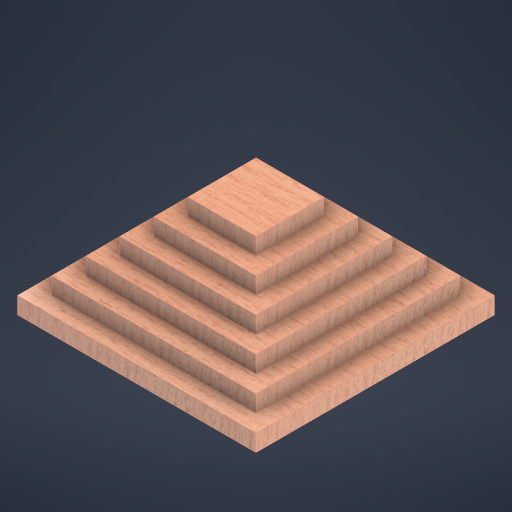
# Autodesk Inventor part: strecha
Saved by Autodesk Inventor 2023 (Build 270158000, 158)
## iProperties
Created: 2022-10-19
Part Number: strecha
Material: Dřevo (dub)
Document SubType Name: Modeling
Designer: zak
Density: 0.76 g/cm^3
Appearance: Dub zimní – přírodní – střední lesk
Mass: 1334.18 g
Surface Area: 1412 cm^2
Volume: 1755.5 cm^3
Author: zak
Autodesk Inventor part; units mm, degrees
ref_plane "YZ Plane" through (0, 0, 0) normal (1, 0, 0) x (0, 1, 0)
ref_plane "XZ Plane" through (0, 0, 0) normal (0, 1, 0) x (-1, 0, 0)
ref_plane "XY Plane" through (0, 0, 0) normal (0, 0, 1) x (1, 0, 0)
sketch "Náčrt1" plane through (0, 0, 0) normal (0, 1, 0) x (-1, 0, 0)
  line L0 (105, 105) -> (-105, 105)
  line L1 (-105, 105) -> (-105, -105)
  line L2 (-105, -105) -> (105, -105)
  line L3 (105, -105) -> (105, 105)
  line L4 (105, 105) -> (-105, -105) construction
  line L5 (-105, 105) -> (105, -105) construction
  point P0 (0, 0)
  dimension "d0" = 210
  dimension "d1" = 210
  constraints: 12 end point, 2 midpoint, 2 parallel, 1 horizontal, 1 perpendicular
  measures "d0" distance of L2.end L1.end
  measures "d1" distance of L1.end L0.end
extrude "Vysunutí1" add sketch "Náčrt1" along normal blind 15
sketch "Náčrt2" plane through (0, 15, 0) normal (0, 1, 0) x (1, 0, 0)
  line L0 (90, -90) -> (-90, -90)
  line L1 (-90, -90) -> (-90, 90)
  line L2 (-90, 90) -> (90, 90)
  line L3 (90, 90) -> (90, -90)
  line L4 (90, -90) -> (-90, 90) construction
  line L5 (-90, -90) -> (90, 90) construction
  point P0 (0, 0)
  dimension "d4" = 180
  dimension "d5" = 180
  constraints: 12 end point, 2 midpoint, 2 parallel, 1 horizontal, 1 perpendicular
  measures "d4" distance of L1.end L2.end
  measures "d5" distance of L0.end L1.end
extrude "Vysunutí2" add sketch "Náčrt2" along normal blind 15
sketch "Náčrt3" plane through (0, 30, 0) normal (0, 1, 0) x (1, 0, 0)
  line L0 (75, -75) -> (-75, -75)
  line L1 (-75, -75) -> (-75, 75)
  line L2 (-75, 75) -> (75, 75)
  line L3 (75, 75) -> (75, -75)
  line L4 (75, -75) -> (-75, 75) construction
  line L5 (-75, -75) -> (75, 75) construction
  point P0 (0, 0)
  dimension "d8" = 150
  dimension "d9" = 150
  constraints: 12 end point, 2 midpoint, 2 parallel, 1 horizontal, 1 perpendicular
  measures "d8" distance of L1.end L2.end
  measures "d9" distance of L0.end L1.end
extrude "Vysunutí3" add sketch "Náčrt3" along normal blind 15
sketch "Náčrt4" plane through (0, 45, 0) normal (0, 1, 0) x (1, 0, 0)
  line L0 (60, -60) -> (-60, -60)
  line L1 (-60, -60) -> (-60, 60)
  line L2 (-60, 60) -> (60, 60)
  line L3 (60, 60) -> (60, -60)
  line L4 (60, -60) -> (-60, 60) construction
  line L5 (-60, -60) -> (60, 60) construction
  point P0 (0, 0)
  dimension "d12" = 120
  dimension "d13" = 120
  constraints: 12 end point, 2 midpoint, 2 parallel, 1 horizontal, 1 perpendicular
  measures "d12" distance of L1.end L2.end
  measures "d13" distance of L0.end L1.end
extrude "Vysunutí4" add sketch "Náčrt4" along normal blind 15
sketch "Náčrt5" plane through (0, 60, 0) normal (0, 1, 0) x (1, 0, 0)
  line L0 (45, -45) -> (-45, -45)
  line L1 (-45, -45) -> (-45, 45)
  line L2 (-45, 45) -> (45, 45)
  line L3 (45, 45) -> (45, -45)
  line L4 (45, -45) -> (-45, 45) construction
  line L5 (-45, -45) -> (45, 45) construction
  point P0 (0, 0)
  dimension "d16" = 90
  dimension "d17" = 90
  constraints: 12 end point, 2 midpoint, 2 parallel, 1 horizontal, 1 perpendicular
  measures "d16" distance of L1.end L2.end
  measures "d17" distance of L0.end L1.end
extrude "Vysunutí5" add sketch "Náčrt5" along normal blind 15
sketch "Náčrt7" plane through (0, 75, 0) normal (0, 1, 0) x (1, 0, 0)
  line L0 (-30, 30) -> (30, 30)
  line L1 (30, 30) -> (30, -30)
  line L2 (30, -30) -> (-30, -30)
  line L3 (-30, -30) -> (-30, 30)
  line L4 (-30, 30) -> (30, -30) construction
  line L5 (30, 30) -> (-30, -30) construction
  point P0 (0, 0)
  dimension "d20" = 60
  dimension "d21" = 60
  constraints: 12 end point, 2 midpoint, 2 parallel, 1 horizontal, 1 perpendicular
  measures "d20" distance of L1.end L2.end
  measures "d21" distance of L0.end L1.end
extrude "Vysunutí6" add sketch "Náčrt7" along normal blind 15
sketch "Náčrt8" plane through (0, 0, 0) normal (0, -1, 0) x (1, 0, 0)
  line L0 (-55, -55) -> (55, -55)
  line L1 (55, -55) -> (55, 55)
  line L2 (55, 55) -> (-55, 55)
  line L3 (-55, 55) -> (-55, -55)
  line L4 (-55, -55) -> (55, 55) construction
  line L5 (55, -55) -> (-55, 55) construction
  point P0 (0, 0)
  dimension "d24" = 110
  dimension "d25" = 110
  constraints: 12 end point, 2 midpoint, 2 parallel, 1 horizontal, 1 perpendicular
  measures "d24" distance of L2.end L1.end
  measures "d25" distance of L0.end L1.end
extrude "Vysunutí7" cut sketch "Náčrt8" against normal blind 10
